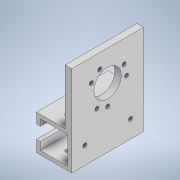
# Autodesk Inventor part: enc holder
Saved by Autodesk Inventor 2022 (Build 260153000, 153)
## iProperties
Created: 2022-05-06
Part Number: enc holder
Material: Generic
Document SubType Name: Modeling
Designer: erasm
Density: 1 g/cm^3
Appearance: Default
Author: erasm
Autodesk Inventor part; units mm, degrees
ref_plane "YZ Plane" through (0, 0, 0) normal (1, 0, 0) x (0, 1, 0)
ref_plane "XZ Plane" through (0, 0, 0) normal (0, 1, 0) x (-1, 0, 0)
ref_plane "XY Plane" through (0, 0, 0) normal (0, 0, 1) x (1, 0, 0)
sketch "Sketch1" plane through (0, 0, 0) normal (0, 0, 1) x (1, 0, 0)
  line L0 (10, 10) -> (-10, 10) construction
  line L1 (-10, 10) -> (-10, -10) construction
  line L2 (-10, -10) -> (10, -10) construction
  line L3 (10, -10) -> (10, 10) construction
  line L4 (-7, -7) -> (-7, 7) construction
  line L5 (-7, 7) -> (7, 7) construction
  line L6 (7, 7) -> (7, -7) construction
  line L7 (7, -7) -> (-7, -7) construction
  line L8 (13.5, 13.5) -> (-13.5, 13.5)
  line L9 (-13.5, 13.5) -> (-13.5, -13.5)
  line L10 (-13.5, -13.5) -> (13.5, -13.5)
  line L11 (13.5, -13.5) -> (13.5, 13.5)
  line L12 (10.5, 10.5) -> (-10.5, 10.5)
  line L13 (-10.5, 10.5) -> (-10.5, -10.5)
  line L14 (-10.5, -10.5) -> (10.5, -10.5)
  line L15 (10.5, -10.5) -> (10.5, 10.5)
  point P0 (0, 0)
  point P1 (-10.5, 0)
  point P2 (0, 10.5)
  dimension "d36" = 21
  dimension "d37" = 21
  dimension "d38" = 3
  dimension "d39" = 3
  dimension "d40" = 3
  dimension "d41" = 3
  constraints: 16 end point, 4 parallel, 2 horizontal, 2 midpoint, 2 perpendicular, 1 horizontal alignment, 1 vertical alignment
  measures "d36" distance of L14.end L13.end
  measures "d37" distance of L13.end L12.end
  measures "d38" distance between parallel lines of L9 L13
  measures "d39" distance between parallel lines of L11 L15
  measures "d40" distance between parallel lines of L8 L12
  measures "d41" distance between parallel lines of L10 L14
extrude "Extrusion1" add sketch "Sketch1" against normal blind 55
sketch "Sketch2" plane through (-13.5, -13.5, 0) normal (-1, 0, 0) x (0, 0, 1)
  line L0 (-80.4804, 19) -> (40.5, 19)
  line L1 (40.5, 19) -> (40.5, 9)
  line L2 (40.5, 9) -> (-80.4804, 9)
  line L3 (-80.4804, 9) -> (-80.4804, 19)
  line L4 (0, 27) -> (-55, 27) projected
  point P0 (0, 13.5)
  dimension "d7" = 10
  dimension "d8" = 8
  constraints: 8 end point, 2 parallel, 1 horizontal, 1 perpendicular
  measures "d7" distance between parallel lines of L2 L0
  measures "d8" distance between parallel lines of L4 L0
extrude "Extrusion2" cut sketch "Sketch2" against normal blind 15.3125
sketch "Sketch3" plane through (-13.5, 13.5, 0) normal (0, 1, 0) x (1, 0, 0)
  line L0 (27, 0) -> (0, 0) projected
  line L1 (3, 55) -> (23, 55) projected
  line L2 (27, 0) -> (22, 0)
  line L3 (22, 0) -> (22, 55)
  line L4 (22, 55) -> (27, 55)
  line L5 (27, 55) -> (27, 0)
  point P0 (13.5, 0)
  dimension "d11" = 5
  constraints: 8 end point, 2 parallel, 1 horizontal, 1 perpendicular, 1 point on line
  measures "d11" distance of L3.end L4.end
extrude "Extrusion3" add sketch "Sketch3" along normal blind 42.3
sketch "Sketch4" plane through (13.5, -13.5, 0) normal (1, 0, 0) x (0, 0, -1)
  line L0 (0, 27) -> (55, 27) projected
  circle A0 centre (27.5, 46) radius 18
  line L1 (0, 69.3) -> (55, 69.3) projected
  circle A1 centre (27.5, 46) radius 3
  point P0 (0, 13.5)
  point P1 (27.5, 69.3)
  dimension "d14" = 36
  dimension "d15" = 19
  dimension "d16" = 6
  constraints: 2 centre point, 1 coincident, 1 midpoint, 1 vertical alignment
  measures "d14" diameter of A0
  measures "d15" distance from line of L0 A0.centre
  measures "d16" diameter of A1
extrude "Extrusion4" cut sketch "Sketch4" against normal blind 42.3 contours A1
sketch "Sketch5" plane through (13.5, -13.5, 0) normal (1, 0, 0) x (0, 0, -1)
  circle A0 centre (27.5, 46) radius 3 projected
  circle A1 centre (27.5, 46) radius 10.5
  point P0 (0, 13.5)
  dimension "d19" = 21
  constraints: 1 centre point, 1 coincident
  measures "d19" diameter of A1
extrude "Extrusion5" cut sketch "Sketch5" against normal blind 42.3
sketch "Sketch6" plane through (13.5, -13.5, 0) normal (1, 0, 0) x (0, 0, -1)
  circle A0 centre (27.5, 30.5) radius 1.5 projected
  circle A1 centre (19.1831, 33.1223) radius 1.495 projected
  circle A2 centre (14.9426, 52.25) radius 1.5 projected
  circle A3 centre (21.372, 58.1415) radius 1.495 projected
  circle A4 centre (40.0574, 52.25) radius 1.5 projected
  circle A5 centre (41.9448, 43.7362) radius 1.495 projected
  point P0 (0, 13.5)
extrude "Extrusion6" cut sketch "Sketch6" against normal blind 42.3
sketch "Sketch7" plane through (13.5, -13.5, 0) normal (1, 0, 0) x (0, 0, -1)
  circle A0 centre (10, 13.5) radius 1.5
  circle A1 centre (45, 13.5) radius 1.5
  line L0 (0, 0) -> (0, 69.3) projected
  line L1 (55, 0) -> (55, 69.3) projected
  point P0 (0, 13.5)
  dimension "d24" = 3
  dimension "d25" = 3
  dimension "d26" = 10
  dimension "d27" = 10
  constraints: 2 centre point, 2 horizontal alignment
  measures "d24" diameter of A0
  measures "d25" diameter of A1
  measures "d26" distance from line of L0 A0.centre
  measures "d27" distance from line of L1 A1.centre
extrude "Extrusion7" cut sketch "Sketch7" against normal blind 10
sketch "Sketch8" plane through (-13.5, -13.5, 0) normal (0, -1, 0) x (1, 0, 0)
  circle A0 centre (13.5, -10) radius 1.5
  circle A1 centre (13.5, -45) radius 1.5
  line L0 (27, -55) -> (0, -55) projected
  line L1 (0, 0) -> (27, 0) projected
  point P0 (13.5, 0)
  point P1 (13.5, 0)
  point P2 (13.5, 0)
  dimension "d30" = 3
  dimension "d31" = 3
  dimension "d32" = 10
  dimension "d33" = 10
  constraints: 2 centre point, 2 midpoint, 2 vertical alignment
  measures "d30" diameter of A0
  measures "d31" diameter of A1
  measures "d32" distance from line of L0 A1.centre
  measures "d33" distance from line of L1 A0.centre
extrude "Extrusion8" cut sketch "Sketch8" against normal through all
body "Solid1"
